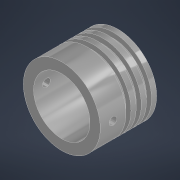
# Autodesk Inventor part: P003-Corps_piston
Saved by Autodesk Inventor 2021.3 (Build 253353000, 353)
## iProperties
Company: HES-SO
Created: 2022-03-18
Part Number: P003-Corps_piston
Material: Aluminium
Document SubType Name: Modeling
Designer: Rémi & Elise
Density: 2.7 g/cm^3
Appearance: Aluminum - Dark
Mass: 21.5358 g
Surface Area: 56.8938 cm^2
Volume: 7.9762 cm^3
Author: Rémi & Elise
Title: Corps piston
Autodesk Inventor part; units mm, degrees
ref_plane "XZ Plane" through (0, 0, 0) normal (0, 1, 0) x (-1, 0, 0)
ref_plane "XY Plane" through (0, 0, 0) normal (0, 0, 1) x (1, 0, 0)
sketch "Sketch5" plane through (0, 0, 0) normal (0, 0, 1) x (1, 0, 0)
  line L0 (-18, 0) -> (3, 0) construction
  line L1 (0, -4.4) -> (0, 26.4) construction
  line L2 (-11, 0) -> (-11, 17)
  line L3 (-11, 17) -> (0, 17)
  line L4 (0, 22) -> (-15, 22)
  line L5 (-15, 22) -> (-15, 20)
  line L6 (-15, 20) -> (-13, 20)
  line L7 (-13, 20) -> (-13, 18)
  line L8 (-13, 18) -> (-15, 18)
  line L9 (-15, 18) -> (-15, 16)
  line L10 (-15, 16) -> (-13, 16)
  line L11 (-13, 16) -> (-13, 14)
  line L12 (-13, 14) -> (-15, 14)
  line L13 (-15, 14) -> (-15, 12)
  line L14 (-15, 12) -> (-13, 12)
  line L15 (0, 22) -> (0, 17)
  line L16 (-13, 12) -> (-13, 10)
  line L17 (-13, 10) -> (-15, 10)
  line L18 (-15, 10) -> (-15, 0)
  line L19 (-15, 0) -> (-11, 0)
  point P0 (0, 0)
  dimension "d18" = 2
  dimension "d34" = 15
  dimension "d35" = 5
  dimension "d38" = 2
  dimension "d39" = 2
  dimension "d40" = 10
  constraints: 36 end point, 11 perpendicular, 10 point on line, 5 parallel, 2 collinear, 2 vertical, 1 horizontal
  measures "d18" distance of L6.end L7.end
  measures "d34" distance of L4.start L4.end
  measures "d35" distance of L4.start L3.end
  measures "d38" distance of L16.end L17.end
  measures "d39" distance between parallel lines of L2 L16
  measures "d40" distance of L17.end L18.end
revolve "Revolution1" add sketch "Sketch5" angle 360 about axis through (0, -10, 0) along (0, 1, 0)
ref_plane "Work Plane1" through (20, 0, 0) normal (1, 0, 0) x (0, 1, 0)
sketch "Sketch6" plane through (20, 0, 0) normal (1, 0, 0) x (0, 1, 0)
  line L0 (12, -15) -> (12, 15) construction
  line L1 (14, -15) -> (14, 15) construction
  line L2 (16, -13) -> (16, 13) construction
  line L3 (16, -15) -> (16, 15) construction
  line L4 (18, -15) -> (18, 15) construction
  line L5 (18, -13) -> (18, 13) construction
  line L6 (20, -13) -> (20, 13) construction
  line L7 (20, -15) -> (20, 15) construction
  line L8 (22, -15) -> (22, 15) construction
  line L9 (-4.4, 0) -> (26.4, 0) construction
  line L10 (0, -15) -> (0, 15) construction
  point P0 (0, 0)
  point P1 (5, -17.5)
  point P2 (5, 17.5)
  point P3 (5, 0)
  dimension "d41" = 5
  constraints: 1 point on line
  measures "d41" distance from line of point (5, 0) L10
hole "Hole1" at (20, 5, 0) direction (-1, 0, 0) diameter 3 end through all
body "Solid3"
